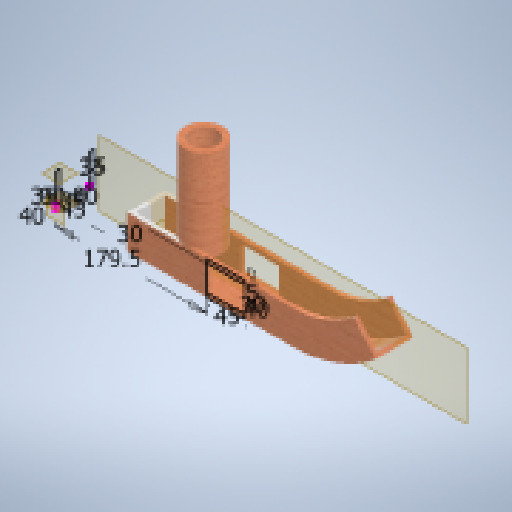
# Autodesk Inventor part: Shooting Ramp
Saved by Autodesk Inventor 2025.2 (Build 292293000, 293)
## iProperties
Created: 2026-04-13
Part Number: Shooting Ramp
Material: Generic
Document SubType Name: Modeling
Designer: abdul
Density: 1 g/cm^3
Appearance: Default
Author: abdul
Autodesk Inventor part; units mm, degrees
ref_plane "YZ Plane" through (0, 0, 0) normal (1, 0, 0) x (0, 1, 0)
ref_plane "XZ Plane" through (0, 0, 0) normal (0, 1, 0) x (-1, 0, 0)
ref_plane "XY Plane" through (0, 0, 0) normal (0, 0, 1) x (1, 0, 0)
sketch "Sketch1" plane through (0, 0, 0) normal (0, 0, 1) x (1, 0, 0)
  line L0 (90, 0) -> (280, 0)
  arc A0 (280, 0) -> (376.4181, 35.0933) centre (280, 150) ccw
  line L1 (280, 0) -> (376.4181, 35.0933) construction
  line L2 (0, 0) -> (0, 82.2351) construction
  dimension "d0" = 150
  dimension "d4" = 20
  dimension "d6" = 280
  dimension "d19" = 173.0413
  dimension "d64" = 90
  constraints: 6 end point, 2 point on circle, 2 vertical, 1 centre point, 1 horizontal, 1 tangent
  measures "d0" radius of A0
  measures "d4" angle of L0 L1
  measures "d6" distance of L2.start L0.end
  measures "d19" distance from line of L2.end L1
  measures "d64" distance from line of L0.start L2
ref_plane "Work Plane1" through (0, 0, 0) normal (1, 0, 0) x (0, 1, 0)
sketch "Sketch2" plane through (0, 0, 0) normal (1, 0, 0) x (0, 1, 0)
  line L0 (0, 0) -> (35, 0)
  line L1 (35, 35) -> (0, 35)
  line L2 (0, 35) -> (0, 0)
  line L3 (35, -5) -> (-5, -5)
  line L4 (-5, -5) -> (-5, 40)
  line L5 (-5, 40) -> (35, 40)
  line L6 (35, -5) -> (35, 0)
  line L7 (35, 35) -> (35, 40)
  dimension "d7" = 35
  dimension "d11" = 35
  dimension "d12" = 90
  dimension "d13" = 35
  dimension "d14" = 40
  dimension "d15" = 45
  dimension "d16" = 35
  constraints: 16 end point, 2 parallel, 1 horizontal, 2 other
  measures "d7" distance of L1.start L1.end
  measures "d11" distance of L1.end L0.start
  measures "d12" angle of L1 L2
  measures "d13" distance from line of L0.end L2
  measures "d14" distance of L4.end L5.end
  measures "d15" distance of L3.end L4.end
  measures "d16" distance from line of L3.start L2
ref_plane "Work Plane4" through (0, -5, 40) normal (0, 0, 1) x (1, 0, 0)
sketch "Sketch3" plane through (0, -5, 40) normal (0, 0, 1) x (1, 0, 0)
  line L0 (179.5, 0) -> (179.5, 40)
  line L1 (179.5, 40) -> (224.5, 40)
  line L2 (224.5, 40) -> (224.5, 0)
  line L3 (224.5, 0) -> (179.5, 0)
  line L4 (179.5, 5) -> (224.5, 5)
  line L5 (179.5, 35) -> (224.5, 35)
  point P0 (0, 5)
  point P1 (0, 0)
  dimension "d20" = 45
  dimension "d21" = 179.5
  dimension "d65" = 40
  dimension "d66" = 30
  dimension "d67" = 5
  dimension "d68" = 30
  constraints: 12 end point, 4 perpendicular, 4 point on line, 1 horizontal
  measures "d20" distance between parallel lines of L2 L0
  measures "d21" distance from line of point (0, 0) L0
  measures "d65" distance of L1.end L2.end
  measures "d66" distance between parallel lines of L5 L4
  measures "d67" distance between parallel lines of L5 L1
  measures "d68" distance from line of point (0, 5) L5
ref_plane "Work Plane6" through (0, 0, 35) normal (0, 1, 0) x (1, 0, 0)
sketch "Sketch4" plane through (0, 0, 35) normal (0, 1, 0) x (1, 0, 0)
  point P0 (0, 35)
ref_plane "Work Plane2" through (224.5, 0, 17.5) normal (0, 0, 1) x (1, 0, 0)
sketch "Sketch5" plane through (224.5, 0, 17.5) normal (0, 0, 1) x (1, 0, 0)
  arc A0 (-77.6803, 0) -> (-64.6037, 0) centre (-71.142, 13.5) ccw
  line L0 (-224.5, 0) -> (-35.51, 0) projected
  line L1 (-224.5, -5) -> (-224.5, 30) projected
  line L2 (-77.6803, 0) -> (-64.6037, 0)
  line L3 (-71.142, -1.5) -> (-71.142, 0)
  dimension "d44" = 30
  dimension "d45" = 13.5
  dimension "d46" = 153.358
  constraints: 4 end point, 3 point on circle, 2 point on line, 1 centre point, 1 collinear, 1 midpoint
  measures "d44" diameter of A0
  measures "d45" distance from line of L0 A0.centre
  measures "d46" distance from line of L1 A0.centre
ref_plane "Work Plane7" through (0, 0, 35) normal (0, 1, 0) x (1, 0, 0)
ref_plane "Work Plane5" through (5, 35, 40) normal (0, 1, 0) x (1, 0, 0)
sketch "Sketch7" plane through (5, 35, 40) normal (0, 1, 0) x (1, 0, 0)
  circle A0 centre (148.3582, 22.5) radius 6.5383
  circle A1 centre (148.3582, 22.5) radius 16
  circle A2 centre (148.3582, 22.5) radius 22.5
  line L0 (-5, 40) -> (-5, 5) projected
  arc A3 (-5, 0) -> (-5, 45) centre (148.3582, 22.5) ccw
  dimension "d48" = 45
  dimension "d49" = 32
  dimension "d55" = 13.0767
  constraints: 4 centre point, 3 coincident, 2 point on circle, 4 other
  measures "d48" diameter of A2
  measures "d49" diameter of A1
  measures "d55" diameter of A0
extrude "Extrusion3" add sketch "Sketch7" along normal blind 100 contours A2
extrude "Extrusion4" add sketch "Sketch7" against normal blind 8 contours A2
ref_plane "Work Plane3" through (90, 0, 0) normal (1, 0, 0) x (0, 1, 0)
sketch "Sketch8" plane through (90, 0, 0) normal (1, 0, 0) x (0, 1, 0)
  line L0 (31.2631, -5) -> (-5, -5) projected
  line L1 (35, -5) -> (-5, -5)
  line L2 (-5, -5) -> (-5, 40)
  line L3 (-5, 40) -> (35, 40)
  line L4 (35, 40) -> (35, 35)
  line L5 (35, 35) -> (0, 35)
  line L6 (0, 35) -> (0, 0)
  line L7 (0, 0) -> (35, 0)
  line L8 (35, 0) -> (35, -5)
  dimension "d59" = 45
  dimension "d60" = 40
  constraints: 16 end point, 7 perpendicular, 1 horizontal, 1 point on line
  measures "d59" distance of L0.end L2.end
  measures "d60" distance between parallel lines of L0 L5
sweep "Sweep3" add profiles "Sketch8" path "Sketch1"
extrude "Extrusion5" cut sketch "Sketch3" against normal through all contours L0 L5 L2 L4
revolve "Revolution2" cut sketch "Sketch5" angle 360 about axis through (153.358, -1.5, 17.5) along (0, 1, 0) picked at (-67.4817, -0.2757) contours L3 L0 A0
sketch "Sketch9" plane through (90, -5, -5) normal (-1, 0, 0) x (0, 0, 1)
  line L0 (0, 40) -> (0, 0)
  line L1 (0, 0) -> (45, 0)
  line L2 (45, 0) -> (45, 40)
  line L3 (45, 40) -> (40, 40)
  line L4 (40, 40) -> (0, 40)
  point P0 (5, 5)
  dimension "d74" = 45
  dimension "d75" = 5
  constraints: 10 end point, 3 perpendicular, 1 collinear
  measures "d74" distance between parallel lines of L0 L2
  measures "d75" distance from line of L3.end L2
extrude "Extrusion6" add sketch "Sketch9" along normal blind 5
body "Solid2"
